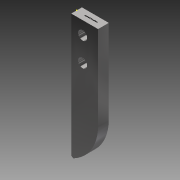
# Autodesk Inventor part: legplate
Saved by Autodesk Inventor 2015 (Build 190159000, 159)
## iProperties
Created: 2020-01-20
Part Number: legplate
Material: Steel, High Strength, Low Alloy
Document SubType Name: Modeling
Designer: hp
Density: 7.85 g/cm^3
Appearance: Steel - Polished
Author: hp
Autodesk Inventor part; units mm, degrees
ref_plane "YZ Plane" through (0, 0, 0) normal (1, 0, 0) x (0, 1, 0)
ref_plane "XZ Plane" through (0, 0, 0) normal (0, 1, 0) x (-1, 0, 0)
ref_plane "XY Plane" through (0, 0, 0) normal (0, 0, 1) x (1, 0, 0)
sketch "Sketch1" plane through (0, 0, 0) normal (1, 0, 0) x (0, 1, 0)
  line L0 (18.6276, 30.145) -> (-681.3735, 30.145)
  line L1 (18.6276, 30.145) -> (18.6276, -29.8549)
  line L2 (18.6276, -29.8549) -> (-681.3735, -29.8549)
  line L3 (-681.3735, -29.8549) -> (-681.3735, 30.145)
  point P0 (0, 0)
  dimension "d0" = 700.0011
  dimension "d1" = 59.9999
  constraints: 8 end point, 2 horizontal, 1 perpendicular, 1 vertical
  measures "d0" distance of L0.start L0.end
  measures "d1" distance of L0.start L1.end
extrude "Extrusion1" add sketch "Sketch1" along normal blind 150
sketch "Sketch2" plane through (0, 18.6276, 30.145) normal (0, 1, 0) x (1, 0, 0)
  line L0 (30.0948, 48.0392) -> (130.9532, 48.0392) construction
  line L1 (130.9532, 48.0392) -> (130.9532, 12.2508) construction
  line L2 (130.9532, 12.2508) -> (30.0948, 12.2508) construction
  line L3 (30.0948, 12.2508) -> (30.0948, 48.0392) construction
  point P0 (0, 30.145)
  constraints: 2 other
fillet "Fillet1" radius 254 1 edges at (150, -681.3735, 0.1451)
chamfer "Chamfer1" distance 12.7 angle 45 1 edges at (0, -681.3735, 0.1451)
sketch "Sketch3" plane through (150, 18.6276, -29.8549) normal (0, 0, -1) x (-1, 0, 0)
  circle A0 centre (86.2337, -73.5365) radius 25.4
  circle A1 centre (86.2337, -207.3813) radius 25.4
  point P0 (150, -18.6276)
  dimension "d8" = 50.8
  dimension "d9" = 50.8
  constraints: 2 centre point
  measures "d8" diameter of A0
  measures "d9" diameter of A1
extrude "Extrusion2" cut sketch "Sketch3" against normal blind 150
body "Solid1"
